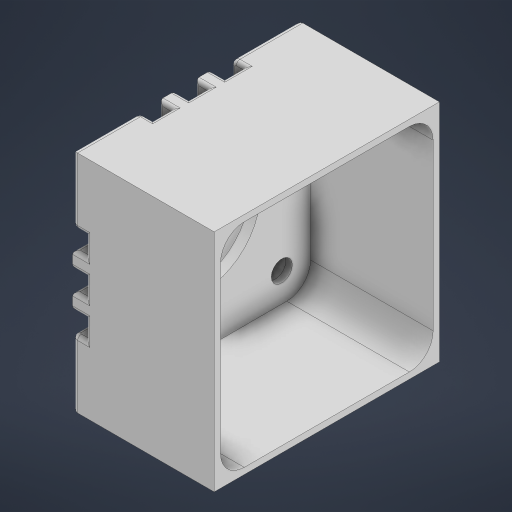
# Autodesk Inventor part: bottom_case
Saved by Autodesk Inventor 2023.1 (Build 271208000, 208)
## iProperties
Created: 2022-11-04
Part Number: bottom_case
Material: Generic
Document SubType Name: Modeling
Designer: amtat
Density: 1 g/cm^3
Appearance: Default
Author: amtat
Autodesk Inventor part; units mm, degrees
ref_plane "YZ Plane" through (0, 0, 0) normal (1, 0, 0) x (0, 1, 0)
ref_plane "XZ Plane" through (0, 0, 0) normal (0, 1, 0) x (-1, 0, 0)
ref_plane "XY Plane" through (0, 0, 0) normal (0, 0, 1) x (1, 0, 0)
sketch "Sketch1" plane through (0, 0, 0) normal (1, 0, 0) x (0, 1, 0)
  line L0 (0, 0) -> (45, 0)
  line L1 (45, 0) -> (45, -45)
  line L2 (45, -45) -> (0, -45)
  line L3 (0, -45) -> (0, 0)
  line L4 (0, 0) -> (22.5, 0)
  line L5 (22.5, 0) -> (22.5, -22.5)
  circle A0 centre (22.5, -22.5) radius 3.5
  line L6 (22.5, -22.5) -> (38, -22.5)
  line L7 (38, -22.5) -> (38, -7)
  circle A1 centre (38, -7) radius 2.1
  circle A2 centre (38, -38) radius 2.1
  circle A3 centre (7, -7) radius 2.1
  circle A4 centre (7, -38) radius 2.1
  dimension "d0" = 45
  dimension "d1" = 45
  dimension "d2" = 22.5
  dimension "d3" = 22.5
  dimension "d4" = 7
  dimension "d5" = 15.5
  dimension "d6" = 15.5
  dimension "d7" = 4.2
  constraints: 16 end point, 5 centre point, 3 perpendicular, 3 symmetric about line, 2 coincident, 2 horizontal, 2 parallel, 1 midpoint, 3 other
  measures "d0" distance of L1.end L2.end
  measures "d1" distance of L0.end L1.end
  measures "d2" distance of L0.start L4.end
  measures "d3" distance of L4.end L5.end
  measures "d4" diameter of A0
  measures "d5" distance of L6.start L6.end
  measures "d6" distance of L6.end L7.end
  measures "d7" diameter of A1
extrude "Extrusion1" add sketch "Sketch1" along normal blind 22.8
sketch "Sketch2" plane through (22.8, 0, 0) normal (1, 0, 0) x (0, 0, -1)
  line L0 (0, 0) -> (45, 0) projected
  line L1 (45, 0) -> (45, 45) projected
  line L2 (45, 45) -> (0, 45) projected
  line L3 (0, 45) -> (0, 0) projected
  circle A0 centre (7, 38) radius 2.1 projected
  circle A1 centre (22.5, 22.5) radius 3.5 projected
  circle A2 centre (38, 38) radius 2.1 projected
  circle A3 centre (7, 7) radius 2.1 projected
  circle A4 centre (38, 7) radius 2.1 projected
  line L4 (45, 45) -> (0, 45) projected
  line L5 (0, 45) -> (1.25, 45)
  line L6 (1.25, 45) -> (1.25, 43.75)
  line L7 (1.25, 43.75) -> (1.25, 1.25)
  line L8 (0, 0) -> (45, 0) projected
  line L9 (1.25, 1.25) -> (43.75, 1.25)
  line L10 (43.75, 1.25) -> (43.75, 43.75)
  line L11 (43.75, 43.75) -> (1.25, 43.75)
  line L12 (43.75, 43.75) -> (39, 43.75)
  line L13 (39, 43.75) -> (39, 39)
  circle A5 centre (39, 39) radius 4.75
  line L14 (22.5, 22.5) -> (29.9927, 22.5)
  line L15 (22.5, 22.5) -> (22.5, 31.435)
  circle A6 centre (39, 6) radius 4.75
  circle A7 centre (6, 39) radius 4.75
  circle A8 centre (6, 6) radius 4.75
  point P0 (6, 43.75)
  point P1 (1.25, 39)
  point P2 (1.25, 6)
  point P3 (6, 1.25)
  point P4 (39, 1.25)
  point P5 (43.75, 6)
  point P6 (43.75, 39)
  dimension "d10" = 1.25
  dimension "d11" = 1.25
  dimension "d12" = 42.5
  dimension "d13" = 42.5
  dimension "d14" = 42.5
  dimension "d15" = 4.75
  dimension "d16" = 4.75
  constraints: 20 end point, 4 perpendicular, 3 centre point, 3 symmetric about line, 2 point on line, 1 coincident, 1 horizontal, 1 parallel, 1 vertical, 6 other
  measures "d10" distance of L2.end L5.end
  measures "d11" distance of L5.end L6.end
  measures "d12" distance of L6.end L7.end
  measures "d13" distance of L7.end L9.end
  measures "d14" distance of L9.end L10.end
  measures "d15" distance of L10.end L12.end
  measures "d16" distance of L12.end L13.end
extrude "Extrusion2" cut sketch "Sketch2" against normal blind 19 contours A7 L11 A5 L10 A6 L9 A8 L7 | A7 | A8 | A5 | A6
sketch "Sketch3" plane through (3.8, 0, 0) normal (1, 0, 0) x (0, 0, -1)
  circle A0 centre (22.5, 22.5) radius 3.5 projected
  circle A1 centre (22.5, 22.5) radius 11.2
  point P0 (0, 0)
  dimension "d19" = 22.4
  constraints: 1 centre point, 1 coincident
  measures "d19" diameter of A1
extrude "Extrusion3" cut sketch "Sketch3" against normal blind 2
sketch "Sketch4" plane through (0, 0, 0) normal (-1, 0, 0) x (0, 0, 1)
  line L0 (0, 0) -> (-45, 0) projected
  line L1 (0, 45) -> (0, 0) projected
  line L2 (-45, 45) -> (0, 45) projected
  line L3 (-45, 0) -> (-45, 45) projected
  circle A0 centre (-7, 38) radius 2.1 projected
  circle A1 centre (-22.5, 22.5) radius 3.5 projected
  circle A2 centre (-38, 38) radius 2.1 projected
  circle A3 centre (-7, 7) radius 2.1 projected
  circle A4 centre (-38, 7) radius 2.1 projected
  circle A5 centre (-7, 7) radius 3.25
  circle A6 centre (-38, 7) radius 3.25
  circle A7 centre (-38, 38) radius 3.25
  circle A8 centre (-7, 38) radius 2.1 projected
  circle A9 centre (-7, 38) radius 3.25
  dimension "d22" = 6.5
  dimension "d23" = 6.5
  dimension "d24" = 6.5
  dimension "d25" = 6.5
  constraints: 4 centre point, 4 coincident
  measures "d22" diameter of A5
  measures "d23" diameter of A6
  measures "d24" diameter of A7
  measures "d25" diameter of A9
extrude "Extrusion4" cut sketch "Sketch4" against normal blind 2.5 contours A5 | A6 | A7 | A9
sketch "Sketch5" plane through (0, 0, 0) normal (-1, 0, 0) x (0, 0, 1)
  circle A0 centre (-7, 38) radius 3.25 projected
  circle A1 centre (-38, 7) radius 3.25 projected
  circle A2 centre (-38, 38) radius 3.25 projected
  circle A3 centre (-7, 7) radius 3.25 projected
  line L0 (0, 0) -> (-45, 0) projected
  line L1 (0, 45) -> (0, 0) projected
  line L2 (-45, 45) -> (0, 45) projected
  line L3 (-45, 0) -> (-45, 45) projected
  circle A4 centre (-22.5, 22.5) radius 3.5 projected
  line L4 (-22.5, 22.5) -> (-45, 22.5)
  line L5 (-45, 22.5) -> (-45, 20.5)
  line L6 (-45, 0) -> (-45, 45) projected
  line L7 (-45, 20.5) -> (-35.5, 20.5)
  line L8 (-35.5, 20.5) -> (-35.5, 24.5)
  line L9 (-35.5, 24.5) -> (-45, 24.5)
  line L10 (-45, 24.5) -> (-45, 20.5)
  line L11 (-45, 20.5) -> (-45, 17.3)
  line L12 (-45, 17.3) -> (-35.5, 17.3)
  line L13 (-35.5, 17.3) -> (-35.5, 13.3)
  line L14 (-35.5, 13.3) -> (-45, 13.3)
  line L15 (-45, 13.3) -> (-45, 17.3)
  line L16 (-45, 24.5) -> (-45, 27.7)
  line L17 (-45, 27.7) -> (-35.5, 27.7)
  line L18 (-35.5, 27.7) -> (-35.5, 31.7)
  line L19 (-35.5, 31.7) -> (-45, 31.7)
  line L20 (-45, 27.7) -> (-45, 31.7)
  line L21 (-22.5, 22.5) -> (-38, 38)
  circle A5 centre (-22.5, 22.5) radius 3.5 projected
  line L22 (-22.5, 22.5) -> (-38, 7)
  line L23 (0, 45) -> (-45, 45)
  line L24 (-20.5, 45) -> (-20.5, 35.5)
  line L25 (-20.5, 35.5) -> (-24.5, 35.5)
  line L26 (-24.5, 35.5) -> (-24.5, 45)
  line L27 (-24.5, 45) -> (-20.5, 45)
  line L28 (-17.3, 45) -> (-17.3, 35.5)
  line L29 (-17.3, 35.5) -> (-13.3, 35.5)
  line L30 (-13.3, 35.5) -> (-13.3, 45)
  line L31 (-13.3, 45) -> (-17.3, 45)
  line L32 (-27.7, 45) -> (-27.7, 35.5)
  line L33 (-27.7, 35.5) -> (-31.7, 35.5)
  line L34 (-31.7, 35.5) -> (-31.7, 45)
  line L35 (0, 0) -> (0, 45)
  line L36 (-45, 0) -> (0, 0)
  line L37 (-24.5, 0) -> (-24.5, 9.5)
  line L38 (-24.5, 9.5) -> (-20.5, 9.5)
  line L39 (-20.5, 9.5) -> (-20.5, 0)
  line L40 (-27.7, 0) -> (-27.7, 9.5)
  line L41 (-27.7, 9.5) -> (-31.7, 9.5)
  line L42 (-31.7, 9.5) -> (-31.7, 0)
  line L43 (-17.3, 0) -> (-17.3, 9.5)
  line L44 (-17.3, 9.5) -> (-13.3, 9.5)
  line L45 (-13.3, 9.5) -> (-13.3, 0)
  line L46 (-9.5, 31.7) -> (0, 31.7)
  line L47 (-9.5, 27.7) -> (-9.5, 31.7)
  line L48 (0, 27.7) -> (-9.5, 27.7)
  line L49 (0, 24.5) -> (-9.5, 24.5)
  line L50 (-9.5, 24.5) -> (-9.5, 20.5)
  line L51 (-9.5, 20.5) -> (0, 20.5)
  line L52 (0, 17.3) -> (-9.5, 17.3)
  line L53 (-9.5, 13.3) -> (0, 13.3)
  line L54 (-9.5, 17.3) -> (-9.5, 13.3)
  dimension "d28" = 2
  dimension "d29" = 9.5
  dimension "d30" = 4
  dimension "d31" = 3.2
  dimension "d32" = 4
  dimension "d33" = 3.2
  dimension "d34" = 4
  constraints: 100 end point, 36 symmetric about line, 14 point on line, 4 horizontal, 4 perpendicular, 2 collinear, 1 midpoint, 1 vertical, 7 other
  measures "d28" distance of L4.end L5.end
  measures "d29" distance of L5.end L7.end
  measures "d30" distance of L7.end L8.end
  measures "d31" distance of L5.end L11.end
  measures "d32" distance of L12.end L13.end
  measures "d33" distance of L9.end L16.end
  measures "d34" distance of L17.end L18.end
extrude "Extrusion5" cut sketch "Sketch5" against normal blind 2.7 contours L0 L43 L44 L45 | L53 L54 L52 L1 | L0 L37 L38 L39 | L51 L50 L49 L1 | L0 L42 L41 L40 | L48 L47 L46 L1 | L3 L12 L13 L14 | L30 L29 L28 L2 | L3 L4 L8 L7 | L24 L25 L26 L2 | L3 L9 L8 L4 | L32 L33 L34 L2 | L3 L19 L18 L17
fillet "Fillet1" radius 1 8 edges at (0, 0, -6.65) (0, 6.65, 0) (0, 0, -38.35) (0, 6.65, -45) (0, 38.35, -45) (0, 38.35, 0) (0, 45, -6.65) (0, 45, -38.35)
fillet "Fillet2" radius 0.75 40 edges at (0.2929, 13.3, -0.2929) (1.85, 13.3, 0) (0, 13.3, -5.25) (0, 15.3, -9.5) (0, 17.3, -4.75) (0, 35.5, -15.3) (0.2929, 44.7071, -13.3) (1.85, 45, -13.3) (0, 39.75, -13.3) (0, 40.25, -17.3) (1.35, 45, -17.3) (2.7, 45, -15.3) (2.7, 45, -22.5) (1.35, 45, -20.5) (0, 40.25, -20.5) (0, 35.5, -22.5) (0, 40.25, -24.5) (1.35, 45, -24.5) (1.35, 45, -27.7) (2.7, 45, -29.7) (1.85, 45, -31.7) (0, 39.75, -31.7) (0.2929, 44.7071, -31.7) (0, 40.25, -27.7) (0, 35.5, -29.7) (2.7, 15.3, 0) (1.35, 17.3, 0) (0, 20.5, -4.75) (1.35, 20.5, 0) (2.7, 22.5, 0) (1.35, 24.5, 0) (0, 24.5, -4.75) (0, 22.5, -9.5) (0, 29.7, -9.5) (0, 27.7, -4.75) (0.2929, 31.7, -0.2929) (1.85, 31.7, 0) (0, 31.7, -5.25) (1.35, 27.7, 0) (2.7, 29.7, 0)
fillet "Fillet3" radius 0.75 40 edges at (0, 9.5, -29.7) (0.2929, 0.2929, -31.7) (1.85, 0, -31.7) (0, 5.25, -31.7) (0, 4.75, -27.7) (2.7, 0, -29.7) (1.35, 0, -27.7) (1.35, 0, -24.5) (2.7, 0, -22.5) (1.35, 0, -20.5) (0, 4.75, -24.5) (0, 9.5, -22.5) (0, 4.75, -20.5) (0, 9.5, -15.3) (0, 4.75, -17.3) (1.35, 0, -17.3) (2.7, 0, -15.3) (0.2929, 0.2929, -13.3) (1.85, 0, -13.3) (0, 5.25, -13.3) (0.2929, 31.7, -44.7071) (1.85, 31.7, -45) (0, 31.7, -39.75) (0, 29.7, -35.5) (0, 27.7, -40.25) (2.7, 29.7, -45) (1.35, 27.7, -45) (0, 24.5, -40.25) (1.35, 24.5, -45) (2.7, 22.5, -45) (0, 20.5, -40.25) (1.35, 20.5, -45) (0, 22.5, -35.5) (0, 17.3, -40.25) (0, 15.3, -35.5) (0.2929, 13.3, -44.7071) (1.85, 13.3, -45) (0, 13.3, -39.75) (1.35, 17.3, -45) (2.7, 15.3, -45)
sketch "Sketch6" plane through (22.8, 0, 0) normal (1, 0, 0) x (0, 0, -1)
  line L0 (1.25, 6) -> (1.25, 39) projected
  arc A0 (6, 43.75) -> (1.25, 39) centre (6, 39) ccw projected
  line L1 (6, 43.75) -> (39, 43.75) projected
  arc A1 (43.75, 39) -> (39, 43.75) centre (39, 39) ccw projected
  line L2 (43.75, 39) -> (43.75, 6) projected
  arc A2 (39, 1.25) -> (43.75, 6) centre (39, 6) ccw projected
  line L3 (39, 1.25) -> (6, 1.25) projected
  arc A3 (1.25, 6) -> (6, 1.25) centre (6, 6) ccw projected
  line L4 (0, 0) -> (45, 0) projected
  line L5 (45, 0) -> (45, 45) projected
  line L6 (45, 45) -> (0, 45) projected
  line L7 (0, 45) -> (0, 0) projected
extrude "Extrusion6" add sketch "Sketch6" along normal blind 5.5
body "Solid1"
